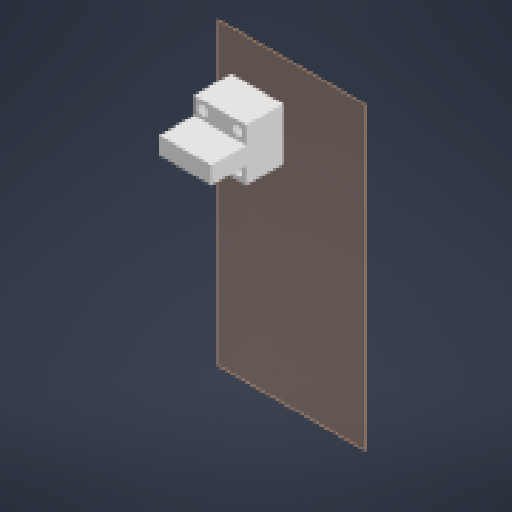
# Autodesk Inventor part: thermoMETER_mount
Saved by Autodesk Inventor 2027 (Build 310192060, 192F)
## iProperties
Created: 2026-05-22
Part Number: thermoMETER_mount
Material: Generic
Document SubType Name: Modeling
Designer: jacob
Density: 1 g/cm^3
Appearance: Default
Author: jacob
Autodesk Inventor part; units mm, degrees
ref_plane "YZ Plane" through (0, 0, 0) normal (1, 0, 0) x (0, 1, 0)
ref_plane "XZ Plane" through (0, 0, 0) normal (0, 1, 0) x (-1, 0, 0)
ref_plane "XY Plane" through (0, 0, 0) normal (0, 0, 1) x (1, 0, 0)
ref_plane "Work Plane4" through (0, 0, 0) normal (0, 0, 1) x (1, 0, 0)
sketch "base_sketch" plane through (0, 0, 0) normal (0, 0, 1) x (1, 0, 0)
  line L0 (-6.25, 78.6816) -> (-43.75, 78.6816)
  line L1 (-43.75, 78.6816) -> (-43.75, 41.1816)
  line L2 (-43.75, 41.1816) -> (-6.25, 41.1816)
  line L3 (-6.25, 41.1816) -> (-6.25, 78.6816)
  circle A0 centre (-12.5, 72.4316) radius 3.25 projected
  circle A1 centre (-12.5, 47.4316) radius 3.25 projected
  circle A2 centre (-37.5, 47.4316) radius 3.25 projected
  circle A3 centre (-37.5, 72.4316) radius 3.25 projected
  point P0 (0, 0)
  dimension "d10" = 6.25
  dimension "d11" = 6.25
  dimension "d12" = 6.25
  dimension "d13" = 6.25
  constraints: 8 end point, 2 parallel, 1 horizontal, 1 perpendicular
  measures "d10" distance from line of A0.centre L0
  measures "d11" distance from line of L2 A1.centre
  measures "d12" distance from line of L1 A2.centre
  measures "d13" distance from line of L3 A1.centre
extrude "base" add sketch "base_sketch" along normal blind 26.8
sketch "label_sketch" plane through (-43.75, 41.1816, 0) normal (-1, 0, 0) x (0, 0, 1)
  line L0 (21.3191, 34.4863) -> (21.3191, -0.1752) construction
  line L1 (21.3191, -0.1752) -> (1.4002, -0.1752) construction
  line L2 (1.4002, -0.1752) -> (1.4002, 34.4863) construction
  line L3 (1.4002, 34.4863) -> (21.3191, 34.4863) construction
  line L4 (18.1353, 33.4662) -> (20.8226, 33.4662)
  line L5 (20.8226, 33.4662) -> (20.8226, 34.4888)
  line L6 (20.8226, 34.4888) -> (21.1833, 34.4888)
  line L7 (21.1833, 34.4888) -> (21.1833, 32.0385)
  line L8 (21.1833, 32.0385) -> (20.8226, 32.0385)
  line L9 (20.8226, 32.0385) -> (20.8226, 33.0611)
  line L10 (20.8226, 33.0611) -> (18.1353, 33.0611)
  line L11 (18.1353, 33.0611) -> (18.1353, 33.4662)
  line L12 (18.1353, 29.9637) -> (18.1353, 30.349)
  line L13 (18.1353, 30.349) -> (19.4394, 30.349)
  spline S0 degree 2 poles (19.4394, 30.349) (19.5975, 30.349) (19.8692, 30.3787) (19.9507, 30.4231) knots 0 0 0 1 2 2 2
  spline S1 degree 2 poles (19.9507, 30.4231) (20.0372, 30.4701) (20.1212, 30.638) (20.1212, 30.7813) knots 0 0 0 1 2 2 2
  spline S2 degree 2 poles (20.1212, 30.7813) (20.1212, 30.9246) (19.968, 31.2284) (19.8445, 31.3741) knots 0 0 0 1 2 2 2
  line L14 (19.8445, 31.3741) -> (18.1353, 31.3741)
  line L15 (18.1353, 31.3741) -> (18.1353, 31.7594)
  line L16 (18.1353, 31.7594) -> (21.3191, 31.7594)
  line L17 (21.3191, 31.7594) -> (21.3191, 31.3741)
  line L18 (21.3191, 31.3741) -> (20.1681, 31.3741)
  spline S3 degree 2 poles (20.1681, 31.3741) (20.3237, 31.2012) (20.4867, 30.8678) (20.4867, 30.68) knots 0 0 0 1 2 2 2
  spline S4 degree 2 poles (20.4867, 30.68) (20.4867, 30.3441) (20.0421, 29.9637) (19.6197, 29.9637) knots 0 0 0 1 2 2 2
  line L19 (19.6197, 29.9637) -> (18.1353, 29.9637)
  spline S5 degree 2 poles (18.0834, 28.4298) (18.0834, 28.9782) (18.6984, 29.5809) (19.2665, 29.5809) knots 0 0 0 1 2 2 2
  spline S6 degree 2 poles (19.2665, 29.5809) (19.8248, 29.5809) (20.4867, 28.9955) (20.4867, 28.5237) knots 0 0 0 1 2 2 2
  spline S7 degree 2 poles (20.4867, 28.5237) (20.4867, 28.3113) (20.3632, 27.9828) (20.2323, 27.8617) knots 0 0 0 1 2 2 2
  spline S8 degree 2 poles (20.2323, 27.8617) (20.1014, 27.7382) (19.7235, 27.6073) (19.4493, 27.6073) knots 0 0 0 1 2 2 2
  line L20 (19.4493, 27.6073) -> (19.2394, 27.6073)
  line L21 (19.2394, 27.6073) -> (19.2394, 29.1906)
  spline S9 degree 2 poles (19.2394, 29.1906) (18.8417, 29.1906) (18.4193, 28.7905) (18.4193, 28.4348) knots 0 0 0 1 2 2 2
  spline S10 degree 2 poles (18.4193, 28.4348) (18.4193, 28.3088) (18.4761, 28.0643) (18.5206, 27.9655) knots 0 0 0 1 2 2 2
  spline S11 degree 2 poles (18.5206, 27.9655) (18.57, 27.8617) (18.6564, 27.7185) (18.696, 27.6716) knots 0 0 0 1 2 2 2
  line L22 (18.696, 27.6716) -> (18.696, 27.6493)
  line L23 (18.696, 27.6493) -> (18.2761, 27.6493)
  spline S12 degree 2 poles (18.2761, 27.6493) (18.2489, 27.716) (18.1698, 27.9186) (18.1476, 27.9976) knots 0 0 0 1 2 2 2
  spline S13 degree 2 poles (18.1476, 27.9976) (18.1155, 28.1087) (18.0834, 28.2915) (18.0834, 28.4298) knots 0 0 0 1 2 2 2
  spline S14 degree 2 poles (19.5333, 27.9828) (19.6889, 27.9877) (19.9161, 28.0519) (19.9927, 28.1137) knots 0 0 0 1 2 2 2
  spline S15 degree 2 poles (19.9927, 28.1137) (20.0792, 28.1804) (20.1706, 28.3903) (20.1706, 28.5459) knots 0 0 0 1 2 2 2
  spline S16 degree 2 poles (20.1706, 28.5459) (20.1706, 28.6991) (20.0792, 28.914) (19.9902, 29.0029) knots 0 0 0 1 2 2 2
  spline S17 degree 2 poles (19.9902, 29.0029) (19.8989, 29.0893) (19.679, 29.1783) (19.5333, 29.1906) knots 0 0 0 1 2 2 2
  line L24 (19.5333, 29.1906) -> (19.5333, 27.9828)
  line L25 (20.01, 26.0043) -> (20.01, 26.024)
  spline S18 degree 2 poles (20.01, 26.024) (20.0224, 26.0685) (20.0273, 26.1648) (20.0273, 26.2315) knots 0 0 0 1 2 2 2
  spline S19 degree 2 poles (20.0273, 26.2315) (20.0273, 26.3871) (19.8914, 26.6934) (19.7581, 26.8317) knots 0 0 0 1 2 2 2
  line L26 (19.7581, 26.8317) -> (18.1353, 26.8317)
  line L27 (18.1353, 26.8317) -> (18.1353, 27.2171)
  line L28 (18.1353, 27.2171) -> (20.4225, 27.2171)
  line L29 (20.4225, 27.2171) -> (20.4225, 26.8317)
  line L30 (20.4225, 26.8317) -> (20.0816, 26.8317)
  spline S20 degree 2 poles (20.0816, 26.8317) (20.2694, 26.6218) (20.4225, 26.3081) (20.4225, 26.1599) knots 0 0 0 1 2 2 2
  spline S21 degree 2 poles (20.4225, 26.1599) (20.4225, 26.1006) (20.4176, 26.0413) (20.4101, 26.0043) knots 0 0 0 1 2 2 2
  line L31 (20.4101, 26.0043) -> (20.01, 26.0043)
  line L32 (18.1353, 23.1119) -> (19.4592, 23.1119)
  spline S22 degree 2 poles (19.4592, 23.1119) (19.6173, 23.1119) (19.8865, 23.1366) (19.9606, 23.1761) knots 0 0 0 1 2 2 2
  spline S23 degree 2 poles (19.9606, 23.1761) (20.0421, 23.2156) (20.1212, 23.3663) (20.1212, 23.4972) knots 0 0 0 1 2 2 2
  spline S24 degree 2 poles (20.1212, 23.4972) (20.1212, 23.6158) (19.9754, 23.8875) (19.8371, 24.0307) knots 0 0 0 1 2 2 2
  spline S25 degree 2 poles (19.8371, 24.0307) (19.8025, 24.0283) (19.7062, 24.0233) (19.642, 24.0233) knots 0 0 0 1 2 2 2
  line L33 (19.642, 24.0233) -> (18.1353, 24.0233)
  line L34 (18.1353, 24.0233) -> (18.1353, 24.4087)
  line L35 (18.1353, 24.4087) -> (19.4592, 24.4087)
  spline S26 degree 2 poles (19.4592, 24.4087) (19.6173, 24.4087) (19.8865, 24.4334) (19.9606, 24.4729) knots 0 0 0 1 2 2 2
  spline S27 degree 2 poles (19.9606, 24.4729) (20.0421, 24.5124) (20.1212, 24.6631) (20.1212, 24.794) knots 0 0 0 1 2 2 2
  spline S28 degree 2 poles (20.1212, 24.794) (20.1212, 24.9175) (19.9655, 25.1917) (19.8445, 25.3201) knots 0 0 0 1 2 2 2
  line L36 (19.8445, 25.3201) -> (18.1353, 25.3201)
  line L37 (18.1353, 25.3201) -> (18.1353, 25.7054)
  line L38 (18.1353, 25.7054) -> (20.4225, 25.7054)
  line L39 (20.4225, 25.7054) -> (20.4225, 25.3201)
  line L40 (20.4225, 25.3201) -> (20.1706, 25.3201)
  spline S29 degree 2 poles (20.1706, 25.3201) (20.3212, 25.1694) (20.4867, 24.873) (20.4867, 24.6952) knots 0 0 0 1 2 2 2
  spline S30 degree 2 poles (20.4867, 24.6952) (20.4867, 24.4926) (20.3015, 24.1789) (20.0915, 24.0974) knots 0 0 0 1 2 2 2
  spline S31 degree 2 poles (20.0915, 24.0974) (20.2866, 23.9221) (20.4867, 23.5911) (20.4867, 23.3984) knots 0 0 0 1 2 2 2
  spline S32 degree 2 poles (20.4867, 23.3984) (20.4867, 23.2502) (20.3953, 23.0082) (20.2916, 22.9192) knots 0 0 0 1 2 2 2
  spline S33 degree 2 poles (20.2916, 22.9192) (20.1878, 22.8278) (19.8766, 22.7266) (19.642, 22.7266) knots 0 0 0 1 2 2 2
  line L41 (19.642, 22.7266) -> (18.1353, 22.7266)
  line L42 (18.1353, 22.7266) -> (18.1353, 23.1119)
  spline S34 degree 2 poles (19.2789, 20.306) (18.7009, 20.306) (18.071, 20.8617) (18.071, 21.3261) knots 0 0 0 1 2 2 2
  spline S35 degree 2 poles (18.071, 21.3261) (18.071, 21.8028) (18.7207, 22.3487) (19.2789, 22.3487) knots 0 0 0 1 2 2 2
  spline S36 degree 2 poles (19.2789, 22.3487) (19.8519, 22.3487) (20.4867, 21.7855) (20.4867, 21.3261) knots 0 0 0 1 2 2 2
  spline S37 degree 2 poles (20.4867, 21.3261) (20.4867, 20.8617) (19.8544, 20.306) (19.2789, 20.306) knots 0 0 0 1 2 2 2
  spline S38 degree 2 poles (19.2789, 20.7036) (19.7235, 20.7036) (20.1557, 21.0272) (20.1557, 21.3261) knots 0 0 0 1 2 2 2
  spline S39 degree 2 poles (20.1557, 21.3261) (20.1557, 21.625) (19.7235, 21.951) (19.2789, 21.951) knots 0 0 0 1 2 2 2
  spline S40 degree 2 poles (19.2789, 21.951) (18.8466, 21.951) (18.402, 21.625) (18.402, 21.3261) knots 0 0 0 1 2 2 2
  spline S41 degree 2 poles (18.402, 21.3261) (18.402, 21.0297) (18.8392, 20.7036) (19.2789, 20.7036) knots 0 0 0 1 2 2 2
  line L43 (18.1353, 17.2678) -> (18.1353, 17.6729)
  line L44 (18.1353, 17.6729) -> (20.7609, 17.6729)
  line L45 (20.7609, 17.6729) -> (18.9751, 18.4683)
  line L46 (18.9751, 18.4683) -> (18.9751, 18.7153)
  line L47 (18.9751, 18.7153) -> (20.7609, 19.5032)
  line L48 (20.7609, 19.5032) -> (18.1353, 19.5032)
  line L49 (18.1353, 19.5032) -> (18.1353, 19.8811)
  line L50 (18.1353, 19.8811) -> (21.1833, 19.8811)
  line L51 (21.1833, 19.8811) -> (21.1833, 19.3278)
  line L52 (21.1833, 19.3278) -> (19.4864, 18.5671)
  line L53 (19.4864, 18.5671) -> (21.1833, 17.831)
  line L54 (21.1833, 17.831) -> (21.1833, 17.2678)
  line L55 (21.1833, 17.2678) -> (18.1353, 17.2678)
  line L56 (18.1353, 16.6503) -> (21.1833, 16.6503)
  line L57 (21.1833, 16.6503) -> (21.1833, 14.7435)
  line L58 (21.1833, 14.7435) -> (20.8226, 14.7435)
  line L59 (20.8226, 14.7435) -> (20.8226, 16.2453)
  line L60 (20.8226, 16.2453) -> (19.9878, 16.2453)
  line L61 (19.9878, 16.2453) -> (19.9878, 14.8448)
  line L62 (19.9878, 14.8448) -> (19.6272, 14.8448)
  line L63 (19.6272, 14.8448) -> (19.6272, 16.2453)
  line L64 (19.6272, 16.2453) -> (18.4959, 16.2453)
  line L65 (18.4959, 16.2453) -> (18.4959, 14.7435)
  line L66 (18.4959, 14.7435) -> (18.1353, 14.7435)
  line L67 (18.1353, 14.7435) -> (18.1353, 16.6503)
  line L68 (18.1353, 13.5875) -> (20.8226, 13.5875)
  line L69 (20.8226, 13.5875) -> (20.8226, 14.6101)
  line L70 (20.8226, 14.6101) -> (21.1833, 14.6101)
  line L71 (21.1833, 14.6101) -> (21.1833, 12.1598)
  line L72 (21.1833, 12.1598) -> (20.8226, 12.1598)
  line L73 (20.8226, 12.1598) -> (20.8226, 13.1824)
  line L74 (20.8226, 13.1824) -> (18.1353, 13.1824)
  line L75 (18.1353, 13.1824) -> (18.1353, 13.5875)
  line L76 (18.1353, 11.8511) -> (21.1833, 11.8511)
  line L77 (21.1833, 11.8511) -> (21.1833, 9.9442)
  line L78 (21.1833, 9.9442) -> (20.8226, 9.9442)
  line L79 (20.8226, 9.9442) -> (20.8226, 11.446)
  line L80 (20.8226, 11.446) -> (19.9878, 11.446)
  line L81 (19.9878, 11.446) -> (19.9878, 10.0455)
  line L82 (19.9878, 10.0455) -> (19.6272, 10.0455)
  line L83 (19.6272, 10.0455) -> (19.6272, 11.446)
  line L84 (19.6272, 11.446) -> (18.4959, 11.446)
  line L85 (18.4959, 11.446) -> (18.4959, 9.9442)
  line L86 (18.4959, 9.9442) -> (18.1353, 9.9442)
  line L87 (18.1353, 9.9442) -> (18.1353, 11.8511)
  line L88 (18.1353, 7.1408) -> (18.1353, 7.6669)
  line L89 (18.1353, 7.6669) -> (19.348, 8.6302)
  line L90 (19.348, 8.6302) -> (19.348, 9.0946)
  line L91 (19.348, 9.0946) -> (18.1353, 9.0946)
  line L92 (18.1353, 9.0946) -> (18.1353, 9.4996)
  line L93 (18.1353, 9.4996) -> (21.1833, 9.4996)
  line L94 (21.1833, 9.4996) -> (21.1833, 8.7142)
  spline S42 degree 2 poles (21.1833, 8.7142) (21.1833, 8.4524) (21.1265, 8.0991) (21.0227, 7.9386) knots 0 0 0 1 2 2 2
  spline S43 degree 2 poles (21.0227, 7.9386) (20.919, 7.778) (20.5954, 7.5928) (20.3558, 7.5928) knots 0 0 0 1 2 2 2
  spline S44 degree 2 poles (20.3558, 7.5928) (20.0224, 7.5928) (19.5703, 7.9337) (19.4617, 8.2251) knots 0 0 0 1 2 2 2
  line L95 (19.4617, 8.2251) -> (18.1353, 7.1408)
  spline S45 degree 2 poles (20.3237, 8.0152) (20.4571, 8.0152) (20.6621, 8.109) (20.7288, 8.2078) knots 0 0 0 1 2 2 2
  spline S46 degree 2 poles (20.7288, 8.2078) (20.7856, 8.2943) (20.8325, 8.524) (20.8325, 8.6919) knots 0 0 0 1 2 2 2
  line L96 (20.8325, 8.6919) -> (20.8325, 9.0946)
  line L97 (20.8325, 9.0946) -> (19.6864, 9.0946)
  line L98 (19.6864, 9.0946) -> (19.6864, 8.7389)
  spline S47 degree 2 poles (19.6864, 8.7389) (19.6864, 8.5635) (19.7482, 8.2844) (19.8445, 8.1881) knots 0 0 0 1 2 2 2
  spline S48 degree 2 poles (19.8445, 8.1881) (19.9285, 8.0991) (20.1656, 8.0152) (20.3237, 8.0152) knots 0 0 0 1 2 2 2
  line L99 (13.1168, 31.6137) -> (14.4407, 31.6137)
  spline S49 degree 2 poles (14.4407, 31.6137) (14.5988, 31.6137) (14.8681, 31.6384) (14.9422, 31.6779) knots 0 0 0 1 2 2 2
  spline S50 degree 2 poles (14.9422, 31.6779) (15.0237, 31.7174) (15.1027, 31.8681) (15.1027, 31.999) knots 0 0 0 1 2 2 2
  spline S51 degree 2 poles (15.1027, 31.999) (15.1027, 32.1176) (14.957, 32.3893) (14.8187, 32.5325) knots 0 0 0 1 2 2 2
  spline S52 degree 2 poles (14.8187, 32.5325) (14.7841, 32.5301) (14.6877, 32.5251) (14.6235, 32.5251) knots 0 0 0 1 2 2 2
  line L100 (14.6235, 32.5251) -> (13.1168, 32.5251)
  line L101 (13.1168, 32.5251) -> (13.1168, 32.9105)
  line L102 (13.1168, 32.9105) -> (14.4407, 32.9105)
  spline S53 degree 2 poles (14.4407, 32.9105) (14.5988, 32.9105) (14.8681, 32.9352) (14.9422, 32.9747) knots 0 0 0 1 2 2 2
  spline S54 degree 2 poles (14.9422, 32.9747) (15.0237, 33.0142) (15.1027, 33.1649) (15.1027, 33.2958) knots 0 0 0 1 2 2 2
  spline S55 degree 2 poles (15.1027, 33.2958) (15.1027, 33.4193) (14.9471, 33.6935) (14.8261, 33.8219) knots 0 0 0 1 2 2 2
  line L103 (14.8261, 33.8219) -> (13.1168, 33.8219)
  line L104 (13.1168, 33.8219) -> (13.1168, 34.2072)
  line L105 (13.1168, 34.2072) -> (15.404, 34.2072)
  line L106 (15.404, 34.2072) -> (15.404, 33.8219)
  line L107 (15.404, 33.8219) -> (15.1521, 33.8219)
  spline S56 degree 2 poles (15.1521, 33.8219) (15.3028, 33.6712) (15.4683, 33.3748) (15.4683, 33.197) knots 0 0 0 1 2 2 2
  spline S57 degree 2 poles (15.4683, 33.197) (15.4683, 32.9944) (15.283, 32.6807) (15.0731, 32.5992) knots 0 0 0 1 2 2 2
  spline S58 degree 2 poles (15.0731, 32.5992) (15.2682, 32.4239) (15.4683, 32.0929) (15.4683, 31.9002) knots 0 0 0 1 2 2 2
  spline S59 degree 2 poles (15.4683, 31.9002) (15.4683, 31.752) (15.3769, 31.51) (15.2731, 31.421) knots 0 0 0 1 2 2 2
  spline S60 degree 2 poles (15.2731, 31.421) (15.1694, 31.3296) (14.8582, 31.2284) (14.6235, 31.2284) knots 0 0 0 1 2 2 2
  line L108 (14.6235, 31.2284) -> (13.1168, 31.2284)
  line L109 (13.1168, 31.2284) -> (13.1168, 31.6137)
  spline S61 degree 2 poles (14.2604, 28.8078) (13.6824, 28.8078) (13.0526, 29.3635) (13.0526, 29.8279) knots 0 0 0 1 2 2 2
  spline S62 degree 2 poles (13.0526, 29.8279) (13.0526, 30.3046) (13.7022, 30.8505) (14.2604, 30.8505) knots 0 0 0 1 2 2 2
  spline S63 degree 2 poles (14.2604, 30.8505) (14.8335, 30.8505) (15.4683, 30.2873) (15.4683, 29.8279) knots 0 0 0 1 2 2 2
  spline S64 degree 2 poles (15.4683, 29.8279) (15.4683, 29.3635) (14.8359, 28.8078) (14.2604, 28.8078) knots 0 0 0 1 2 2 2
  spline S65 degree 2 poles (14.2604, 29.2054) (14.705, 29.2054) (15.1373, 29.529) (15.1373, 29.8279) knots 0 0 0 1 2 2 2
  spline S66 degree 2 poles (15.1373, 29.8279) (15.1373, 30.1267) (14.705, 30.4528) (14.2604, 30.4528) knots 0 0 0 1 2 2 2
  spline S67 degree 2 poles (14.2604, 30.4528) (13.8282, 30.4528) (13.3836, 30.1267) (13.3836, 29.8279) knots 0 0 0 1 2 2 2
  spline S68 degree 2 poles (13.3836, 29.8279) (13.3836, 29.5315) (13.8208, 29.2054) (14.2604, 29.2054) knots 0 0 0 1 2 2 2
  line L110 (13.1168, 26.6341) -> (13.1168, 27.0195)
  line L111 (13.1168, 27.0195) -> (13.3688, 27.0195)
  spline S69 degree 2 poles (13.3688, 27.0195) (13.2131, 27.1973) (13.0526, 27.5159) (13.0526, 27.7135) knots 0 0 0 1 2 2 2
  spline S70 degree 2 poles (13.0526, 27.7135) (13.0526, 27.8617) (13.1514, 28.126) (13.2576, 28.2224) knots 0 0 0 1 2 2 2
  spline S71 degree 2 poles (13.2576, 28.2224) (13.3638, 28.3212) (13.6874, 28.4298) (13.9196, 28.4298) knots 0 0 0 1 2 2 2
  line L112 (13.9196, 28.4298) -> (15.404, 28.4298)
  line L113 (15.404, 28.4298) -> (15.404, 28.0445)
  line L114 (15.404, 28.0445) -> (14.0999, 28.0445)
  spline S72 degree 2 poles (14.0999, 28.0445) (13.9171, 28.0445) (13.6775, 28.0174) (13.5886, 27.9704) knots 0 0 0 1 2 2 2
  spline S73 degree 2 poles (13.5886, 27.9704) (13.4997, 27.9235) (13.4182, 27.7629) (13.4182, 27.6123) knots 0 0 0 1 2 2 2
  spline S74 degree 2 poles (13.4182, 27.6123) (13.4182, 27.4715) (13.5787, 27.1528) (13.6948, 27.0195) knots 0 0 0 1 2 2 2
  line L115 (13.6948, 27.0195) -> (15.404, 27.0195)
  line L116 (15.404, 27.0195) -> (15.404, 26.6341)
  line L117 (15.404, 26.6341) -> (13.1168, 26.6341)
  line L118 (13.1168, 24.2802) -> (13.1168, 24.6655)
  line L119 (13.1168, 24.6655) -> (14.421, 24.6655)
  spline S75 degree 2 poles (14.421, 24.6655) (14.5791, 24.6655) (14.8508, 24.6952) (14.9323, 24.7396) knots 0 0 0 1 2 2 2
  spline S76 degree 2 poles (14.9323, 24.7396) (15.0187, 24.7866) (15.1027, 24.9545) (15.1027, 25.0978) knots 0 0 0 1 2 2 2
  spline S77 degree 2 poles (15.1027, 25.0978) (15.1027, 25.2411) (14.9496, 25.5449) (14.8261, 25.6906) knots 0 0 0 1 2 2 2
  line L120 (14.8261, 25.6906) -> (13.1168, 25.6906)
  line L121 (13.1168, 25.6906) -> (13.1168, 26.0759)
  line L122 (13.1168, 26.0759) -> (15.404, 26.0759)
  line L123 (15.404, 26.0759) -> (15.404, 25.6906)
  line L124 (15.404, 25.6906) -> (15.1496, 25.6906)
  spline S78 degree 2 poles (15.1496, 25.6906) (15.3052, 25.5177) (15.4683, 25.1842) (15.4683, 24.9965) knots 0 0 0 1 2 2 2
  spline S79 degree 2 poles (15.4683, 24.9965) (15.4683, 24.6606) (15.0237, 24.2802) (14.6013, 24.2802) knots 0 0 0 1 2 2 2
  line L125 (14.6013, 24.2802) -> (13.1168, 24.2802)
  spline S80 degree 2 poles (13.0724, 23.0477) (13.0724, 23.3614) (13.4305, 23.7146) (13.8183, 23.7146) knots 0 0 0 1 2 2 2
  line L126 (13.8183, 23.7146) -> (15.0854, 23.7146)
  line L127 (15.0854, 23.7146) -> (15.0854, 23.9739)
  line L128 (15.0854, 23.9739) -> (15.404, 23.9739)
  line L129 (15.404, 23.9739) -> (15.404, 23.7146)
  line L130 (15.404, 23.7146) -> (16.0611, 23.7146)
  line L131 (16.0611, 23.7146) -> (16.0611, 23.3293)
  line L132 (16.0611, 23.3293) -> (15.404, 23.3293)
  line L133 (15.404, 23.3293) -> (15.404, 22.6204)
  line L134 (15.404, 22.6204) -> (15.0854, 22.6204)
  line L135 (15.0854, 22.6204) -> (15.0854, 23.3293)
  line L136 (15.0854, 23.3293) -> (13.9961, 23.3293)
  spline S81 degree 2 poles (13.9961, 23.3293) (13.8232, 23.3293) (13.633, 23.3169) (13.5515, 23.2749) knots 0 0 0 1 2 2 2
  spline S82 degree 2 poles (13.5515, 23.2749) (13.4799, 23.2403) (13.4083, 23.0847) (13.4083, 22.9513) knots 0 0 0 1 2 2 2
  spline S83 degree 2 poles (13.4083, 22.9513) (13.4083, 22.8575) (13.4651, 22.6821) (13.4824, 22.6426) knots 0 0 0 1 2 2 2
  line L137 (13.4824, 22.6426) -> (13.4824, 22.6204)
  line L138 (13.4824, 22.6204) -> (13.1366, 22.6204)
  spline S84 degree 2 poles (13.1366, 22.6204) (13.1069, 22.729) (13.0724, 22.9513) (13.0724, 23.0477) knots 0 0 0 1 2 2 2
  spline S85 degree 2 poles (14.1048, 19.1574) (13.8702, 19.1574) (13.4725, 19.313) (13.3391, 19.4439) knots 0 0 0 1 2 2 2
  spline S86 degree 2 poles (13.3391, 19.4439) (13.1983, 19.5798) (13.0526, 19.9206) (13.0526, 20.1257) knots 0 0 0 1 2 2 2
  spline S87 degree 2 poles (13.0526, 20.1257) (13.0526, 20.3307) (13.1909, 20.6691) (13.3292, 20.7975) knots 0 0 0 1 2 2 2
  spline S88 degree 2 poles (13.3292, 20.7975) (13.4947, 20.9556) (14.0505, 21.1334) (14.4556, 21.1334) knots 0 0 0 1 2 2 2
  spline S89 degree 2 poles (14.4556, 21.1334) (14.8532, 21.1334) (15.493, 20.9704) (15.7301, 20.8) knots 0 0 0 1 2 2 2
  spline S90 degree 2 poles (15.7301, 20.8) (15.9623, 20.6345) (16.2216, 20.1108) (16.2216, 19.7675) knots 0 0 0 1 2 2 2
  spline S91 degree 2 poles (16.2216, 19.7675) (16.2216, 19.6662) (16.2019, 19.4884) (16.1796, 19.4217) knots 0 0 0 1 2 2 2
  line L139 (16.1796, 19.4217) -> (15.7869, 19.4217)
  line L140 (15.7869, 19.4217) -> (15.7869, 19.439)
  spline S92 degree 2 poles (15.7869, 19.439) (15.8165, 19.4958) (15.8684, 19.7033) (15.8684, 19.8218) knots 0 0 0 1 2 2 2
  spline S93 degree 2 poles (15.8684, 19.8218) (15.8684, 20.2022) (15.3546, 20.6691) (14.8508, 20.7135) knots 0 0 0 1 2 2 2
  spline S94 degree 2 poles (14.8508, 20.7135) (14.952, 20.5678) (15.0632, 20.2615) (15.0632, 20.0787) knots 0 0 0 1 2 2 2
  spline S95 degree 2 poles (15.0632, 20.0787) (15.0632, 19.9009) (14.9916, 19.6341) (14.8829, 19.4884) knots 0 0 0 1 2 2 2
  spline S96 degree 2 poles (14.8829, 19.4884) (14.7569, 19.3204) (14.3666, 19.1574) (14.1048, 19.1574) knots 0 0 0 1 2 2 2
  spline S97 degree 2 poles (14.0875, 19.5724) (14.2752, 19.5724) (14.5297, 19.6712) (14.6186, 19.7798) knots 0 0 0 1 2 2 2
  spline S98 degree 2 poles (14.6186, 19.7798) (14.6828, 19.8614) (14.7248, 20.0639) (14.7248, 20.1701) knots 0 0 0 1 2 2 2
  spline S99 degree 2 poles (14.7248, 20.1701) (14.7248, 20.3134) (14.6383, 20.5826) (14.5568, 20.7135) knots 0 0 0 1 2 2 2
  spline S100 degree 2 poles (14.5568, 20.7135) (14.5124, 20.716) (14.4284, 20.7209) (14.3642, 20.7209) knots 0 0 0 1 2 2 2
  spline S101 degree 2 poles (14.3642, 20.7209) (14.048, 20.7209) (13.6602, 20.5974) (13.5589, 20.5036) knots 0 0 0 1 2 2 2
  spline S102 degree 2 poles (13.5589, 20.5036) (13.4626, 20.4171) (13.386, 20.2294) (13.386, 20.1232) knots 0 0 0 1 2 2 2
  spline S103 degree 2 poles (13.386, 20.1232) (13.386, 19.8762) (13.7368, 19.5724) (14.0875, 19.5724) knots 0 0 0 1 2 2 2
  line L141 (16.3007, 17.5297) -> (12.4548, 18.7227)
  line L142 (12.4548, 18.7227) -> (12.4548, 19.0685)
  line L143 (12.4548, 19.0685) -> (16.3007, 17.8804)
  line L144 (16.3007, 17.8804) -> (16.3007, 17.5297)
  line L145 (13.1168, 15.3141) -> (13.1168, 17.1937)
  line L146 (13.1168, 17.1937) -> (13.5491, 17.1937)
  spline S104 degree 2 poles (13.5491, 17.1937) (13.7393, 16.9912) (14.0925, 16.6306) (14.2827, 16.4577) knots 0 0 0 1 2 2 2
  spline S105 degree 2 poles (14.2827, 16.4577) (14.6655, 16.1094) (15.1249, 15.855) (15.3695, 15.855) knots 0 0 0 1 2 2 2
  spline S106 degree 2 poles (15.3695, 15.855) (15.4979, 15.855) (15.6906, 15.934) (15.7523, 16.0057) knots 0 0 0 1 2 2 2
  spline S107 degree 2 poles (15.7523, 16.0057) (15.8141, 16.0773) (15.8758, 16.265) (15.8758, 16.3786) knots 0 0 0 1 2 2 2
  spline S108 degree 2 poles (15.8758, 16.3786) (15.8758, 16.4873) (15.8215, 16.7096) (15.7795, 16.8109) knots 0 0 0 1 2 2 2
  spline S109 degree 2 poles (15.7795, 16.8109) (15.7449, 16.8973) (15.6461, 17.0579) (15.6115, 17.1073) knots 0 0 0 1 2 2 2
  line L147 (15.6115, 17.1073) -> (15.6115, 17.1295)
  line L148 (15.6115, 17.1295) -> (16.0463, 17.1295)
  spline S110 degree 2 poles (16.0463, 17.1295) (16.108, 17.0036) (16.229, 16.5515) (16.229, 16.349) knots 0 0 0 1 2 2 2
  spline S111 degree 2 poles (16.229, 16.349) (16.229, 15.9217) (15.777, 15.44) (15.3917, 15.44) knots 0 0 0 1 2 2 2
  spline S112 degree 2 poles (15.3917, 15.44) (15.2114, 15.44) (14.91, 15.524) (14.7816, 15.5981) knots 0 0 0 1 2 2 2
  spline S113 degree 2 poles (14.7816, 15.5981) (14.6482, 15.6722) (14.3864, 15.8871) (14.2604, 16.0057) knots 0 0 0 1 2 2 2
  spline S114 degree 2 poles (14.2604, 16.0057) (14.0505, 16.1983) (13.6009, 16.6701) (13.47, 16.8109) knots 0 0 0 1 2 2 2
  line L149 (13.47, 16.8109) -> (13.47, 15.3141)
  line L150 (13.47, 15.3141) -> (13.1168, 15.3141)
  line L151 (14.1641, 12.9453) -> (14.1641, 13.3084)
  line L152 (14.1641, 13.3084) -> (13.1168, 13.3084)
  line L153 (13.1168, 13.3084) -> (13.1168, 13.7011)
  line L154 (13.1168, 13.7011) -> (14.1641, 13.7011)
  line L155 (14.1641, 13.7011) -> (14.1641, 15.0473)
  line L156 (14.1641, 15.0473) -> (14.5939, 15.0473)
  line L157 (14.5939, 15.0473) -> (16.1648, 13.6838)
  line L158 (16.1648, 13.6838) -> (16.1648, 13.3084)
  line L159 (16.1648, 13.3084) -> (14.4926, 13.3084)
  line L160 (14.4926, 13.3084) -> (14.4926, 12.9453)
  line L161 (14.4926, 12.9453) -> (14.1641, 12.9453)
  line L162 (14.4926, 13.7011) -> (15.6832, 13.7011)
  line L163 (15.6832, 13.7011) -> (14.4926, 14.7262)
  line L164 (14.4926, 14.7262) -> (14.4926, 13.7011)
  line L165 (16.3007, 11.3522) -> (12.4548, 12.5452)
  line L166 (12.4548, 12.5452) -> (12.4548, 12.891)
  line L167 (12.4548, 12.891) -> (16.3007, 11.7029)
  line L168 (16.3007, 11.7029) -> (16.3007, 11.3522)
  line L169 (13.1168, 9.1365) -> (13.1168, 11.0162)
  line L170 (13.1168, 11.0162) -> (13.5491, 11.0162)
  spline S115 degree 2 poles (13.5491, 11.0162) (13.7393, 10.8137) (14.0925, 10.4531) (14.2827, 10.2802) knots 0 0 0 1 2 2 2
  spline S116 degree 2 poles (14.2827, 10.2802) (14.6655, 9.9319) (15.1249, 9.6775) (15.3695, 9.6775) knots 0 0 0 1 2 2 2
  spline S117 degree 2 poles (15.3695, 9.6775) (15.4979, 9.6775) (15.6906, 9.7565) (15.7523, 9.8282) knots 0 0 0 1 2 2 2
  spline S118 degree 2 poles (15.7523, 9.8282) (15.8141, 9.8998) (15.8758, 10.0875) (15.8758, 10.2011) knots 0 0 0 1 2 2 2
  spline S119 degree 2 poles (15.8758, 10.2011) (15.8758, 10.3098) (15.8215, 10.5321) (15.7795, 10.6334) knots 0 0 0 1 2 2 2
  spline S120 degree 2 poles (15.7795, 10.6334) (15.7449, 10.7198) (15.6461, 10.8804) (15.6115, 10.9298) knots 0 0 0 1 2 2 2
  line L171 (15.6115, 10.9298) -> (15.6115, 10.952)
  line L172 (15.6115, 10.952) -> (16.0463, 10.952)
  spline S121 degree 2 poles (16.0463, 10.952) (16.108, 10.826) (16.229, 10.374) (16.229, 10.1715) knots 0 0 0 1 2 2 2
  spline S122 degree 2 poles (16.229, 10.1715) (16.229, 9.7442) (15.777, 9.2625) (15.3917, 9.2625) knots 0 0 0 1 2 2 2
  spline S123 degree 2 poles (15.3917, 9.2625) (15.2114, 9.2625) (14.91, 9.3465) (14.7816, 9.4206) knots 0 0 0 1 2 2 2
  spline S124 degree 2 poles (14.7816, 9.4206) (14.6482, 9.4947) (14.3864, 9.7096) (14.2604, 9.8282) knots 0 0 0 1 2 2 2
  spline S125 degree 2 poles (14.2604, 9.8282) (14.0505, 10.0208) (13.6009, 10.4926) (13.47, 10.6334) knots 0 0 0 1 2 2 2
  line L173 (13.47, 10.6334) -> (13.47, 9.1365)
  line L174 (13.47, 9.1365) -> (13.1168, 9.1365)
  spline S126 degree 2 poles (14.6408, 6.832) (13.8208, 6.832) (13.0526, 7.3087) (13.0526, 7.8052) knots 0 0 0 1 2 2 2
  spline S127 degree 2 poles (13.0526, 7.8052) (13.0526, 8.3091) (13.8356, 8.7809) (14.6383, 8.7809) knots 0 0 0 1 2 2 2
  spline S128 degree 2 poles (14.6383, 8.7809) (15.4633, 8.7809) (16.2266, 8.3042) (16.2266, 7.8052) knots 0 0 0 1 2 2 2
  spline S129 degree 2 poles (16.2266, 7.8052) (16.2266, 7.3038) (15.4362, 6.832) (14.6408, 6.832) knots 0 0 0 1 2 2 2
  spline S130 degree 2 poles (13.7121, 7.3557) (13.8628, 7.2964) (14.3271, 7.247) (14.6408, 7.247) knots 0 0 0 1 2 2 2
  spline S131 degree 2 poles (14.6408, 7.247) (14.9545, 7.247) (15.4164, 7.2964) (15.572, 7.3581) knots 0 0 0 1 2 2 2
  spline S132 degree 2 poles (15.572, 7.3581) (15.7276, 7.4199) (15.8882, 7.6348) (15.8882, 7.8052) knots 0 0 0 1 2 2 2
  spline S133 degree 2 poles (15.8882, 7.8052) (15.8882, 7.9756) (15.7276, 8.1955) (15.5671, 8.2597) knots 0 0 0 1 2 2 2
  spline S134 degree 2 poles (15.5671, 8.2597) (15.4115, 8.3214) (14.9372, 8.3659) (14.6383, 8.3659) knots 0 0 0 1 2 2 2
  spline S135 degree 2 poles (14.6383, 8.3659) (14.3172, 8.3659) (13.8875, 8.3264) (13.7195, 8.2622) knots 0 0 0 1 2 2 2
  spline S136 degree 2 poles (13.7195, 8.2622) (13.5614, 8.2029) (13.391, 7.9831) (13.391, 7.8052) knots 0 0 0 1 2 2 2
  spline S137 degree 2 poles (13.391, 7.8052) (13.391, 7.6372) (13.5515, 7.4174) (13.7121, 7.3557) knots 0 0 0 1 2 2 2
  line L175 (13.1168, 4.5621) -> (13.1168, 6.4418)
  line L176 (13.1168, 6.4418) -> (13.5491, 6.4418)
  spline S138 degree 2 poles (13.5491, 6.4418) (13.7393, 6.2392) (14.0925, 5.8786) (14.2827, 5.7057) knots 0 0 0 1 2 2 2
  spline S139 degree 2 poles (14.2827, 5.7057) (14.6655, 5.3574) (15.1249, 5.103) (15.3695, 5.103) knots 0 0 0 1 2 2 2
  spline S140 degree 2 poles (15.3695, 5.103) (15.4979, 5.103) (15.6906, 5.1821) (15.7523, 5.2537) knots 0 0 0 1 2 2 2
  spline S141 degree 2 poles (15.7523, 5.2537) (15.8141, 5.3253) (15.8758, 5.513) (15.8758, 5.6267) knots 0 0 0 1 2 2 2
  spline S142 degree 2 poles (15.8758, 5.6267) (15.8758, 5.7353) (15.8215, 5.9576) (15.7795, 6.0589) knots 0 0 0 1 2 2 2
  spline S143 degree 2 poles (15.7795, 6.0589) (15.7449, 6.1454) (15.6461, 6.3059) (15.6115, 6.3553) knots 0 0 0 1 2 2 2
  line L177 (15.6115, 6.3553) -> (15.6115, 6.3775)
  line L178 (15.6115, 6.3775) -> (16.0463, 6.3775)
  spline S144 degree 2 poles (16.0463, 6.3775) (16.108, 6.2516) (16.229, 5.7996) (16.229, 5.597) knots 0 0 0 1 2 2 2
  spline S145 degree 2 poles (16.229, 5.597) (16.229, 5.1697) (15.777, 4.688) (15.3917, 4.688) knots 0 0 0 1 2 2 2
  spline S146 degree 2 poles (15.3917, 4.688) (15.2114, 4.688) (14.91, 4.772) (14.7816, 4.8461) knots 0 0 0 1 2 2 2
  spline S147 degree 2 poles (14.7816, 4.8461) (14.6482, 4.9202) (14.3864, 5.1351) (14.2604, 5.2537) knots 0 0 0 1 2 2 2
  spline S148 degree 2 poles (14.2604, 5.2537) (14.0505, 5.4463) (13.6009, 5.9181) (13.47, 6.0589) knots 0 0 0 1 2 2 2
  line L179 (13.47, 6.0589) -> (13.47, 4.5621)
  line L180 (13.47, 4.5621) -> (13.1168, 4.5621)
  spline S149 degree 2 poles (14.1048, 2.2279) (13.8702, 2.2279) (13.4725, 2.3835) (13.3391, 2.5144) knots 0 0 0 1 2 2 2
  spline S150 degree 2 poles (13.3391, 2.5144) (13.1983, 2.6503) (13.0526, 2.9911) (13.0526, 3.1962) knots 0 0 0 1 2 2 2
  spline S151 degree 2 poles (13.0526, 3.1962) (13.0526, 3.4012) (13.1909, 3.7396) (13.3292, 3.868) knots 0 0 0 1 2 2 2
  spline S152 degree 2 poles (13.3292, 3.868) (13.4947, 4.0261) (14.0505, 4.2039) (14.4556, 4.2039) knots 0 0 0 1 2 2 2
  spline S153 degree 2 poles (14.4556, 4.2039) (14.8532, 4.2039) (15.493, 4.0409) (15.7301, 3.8705) knots 0 0 0 1 2 2 2
  spline S154 degree 2 poles (15.7301, 3.8705) (15.9623, 3.705) (16.2216, 3.1813) (16.2216, 2.838) knots 0 0 0 1 2 2 2
  spline S155 degree 2 poles (16.2216, 2.838) (16.2216, 2.7367) (16.2019, 2.5589) (16.1796, 2.4922) knots 0 0 0 1 2 2 2
  line L181 (16.1796, 2.4922) -> (15.7869, 2.4922)
  line L182 (15.7869, 2.4922) -> (15.7869, 2.5095)
  spline S156 degree 2 poles (15.7869, 2.5095) (15.8165, 2.5663) (15.8684, 2.7738) (15.8684, 2.8923) knots 0 0 0 1 2 2 2
  spline S157 degree 2 poles (15.8684, 2.8923) (15.8684, 3.2727) (15.3546, 3.7396) (14.8508, 3.784) knots 0 0 0 1 2 2 2
  spline S158 degree 2 poles (14.8508, 3.784) (14.952, 3.6383) (15.0632, 3.332) (15.0632, 3.1492) knots 0 0 0 1 2 2 2
  spline S159 degree 2 poles (15.0632, 3.1492) (15.0632, 2.9714) (14.9916, 2.7046) (14.8829, 2.5589) knots 0 0 0 1 2 2 2
  spline S160 degree 2 poles (14.8829, 2.5589) (14.7569, 2.3909) (14.3666, 2.2279) (14.1048, 2.2279) knots 0 0 0 1 2 2 2
  spline S161 degree 2 poles (14.0875, 2.6429) (14.2752, 2.6429) (14.5297, 2.7417) (14.6186, 2.8504) knots 0 0 0 1 2 2 2
  spline S162 degree 2 poles (14.6186, 2.8504) (14.6828, 2.9319) (14.7248, 3.1344) (14.7248, 3.2406) knots 0 0 0 1 2 2 2
  spline S163 degree 2 poles (14.7248, 3.2406) (14.7248, 3.3839) (14.6383, 3.6531) (14.5568, 3.784) knots 0 0 0 1 2 2 2
  spline S164 degree 2 poles (14.5568, 3.784) (14.5124, 3.7865) (14.4284, 3.7914) (14.3642, 3.7914) knots 0 0 0 1 2 2 2
  spline S165 degree 2 poles (14.3642, 3.7914) (14.048, 3.7914) (13.6602, 3.6679) (13.5589, 3.5741) knots 0 0 0 1 2 2 2
  spline S166 degree 2 poles (13.5589, 3.5741) (13.4626, 3.4876) (13.386, 3.2999) (13.386, 3.1937) knots 0 0 0 1 2 2 2
  spline S167 degree 2 poles (13.386, 3.1937) (13.386, 2.9467) (13.7368, 2.6429) (14.0875, 2.6429) knots 0 0 0 1 2 2 2
  point P0 (0, -41.1816)
  constraints: 2 other
extrude "label" cut sketch "label_sketch" against normal blind 1
sketch "top_sketch" plane through (0, 0, 26.8) normal (0, 0, 1) x (1, 0, 0)
  line L0 (-43.75, 66.1816) -> (-6.25, 66.1816)
  line L1 (-6.25, 53.6816) -> (-43.75, 53.6816)
  line L2 (-6.25, 66.1816) -> (-6.25, 53.6816)
  line L3 (-6.25, 41.1816) -> (-6.25, 78.6816)
  line L4 (-43.75, 53.6816) -> (-43.75, 66.1816)
  line L5 (-43.75, 41.1816) -> (-6.25, 41.1816) projected
  line L6 (-25, 66.1816) -> (-25, 78.6816)
  line L7 (-6.25, 78.6816) -> (-43.75, 78.6816) projected
  line L8 (-25, 53.6816) -> (-25, 41.1816)
  point P0 (0, 0)
  dimension "d21" = 12.5
  constraints: 14 end point, 4 midpoint, 2 collinear, 1 parallel
  measures "d21" distance between parallel lines of L0 L1
extrude "top" add sketch "top_sketch" along normal blind 25 contours L0 L2 L1 L4
equation "\"d11\" = d10"
equation "\"d12\" = d10"
equation "\"d13\" = d10"
body "Solid2"
